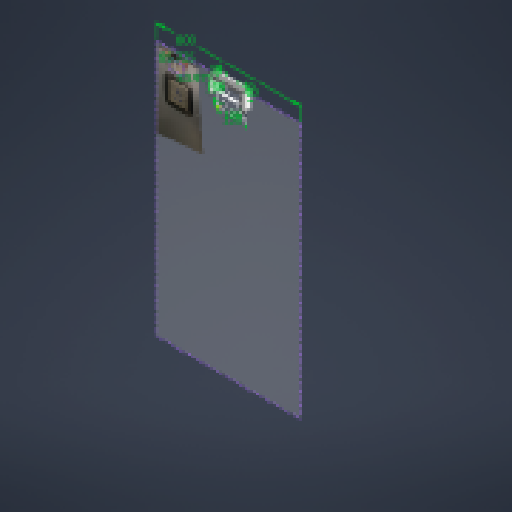
# Autodesk Inventor part: DoorButtonMount
Saved by Autodesk Inventor 2023 (Build 270158000, 158)
## iProperties
Created: 2023-12-06
Part Number: DoorButtonMount
Material: Generic
Document SubType Name: Modeling
Designer: FizzyApple12
Density: 1 g/cm^3
Appearance: Default
Author: FizzyApple12
Autodesk Inventor part; units mm, degrees
ref_plane "YZ Plane" through (0, 0, 0) normal (1, 0, 0) x (0, 1, 0)
ref_plane "XZ Plane" through (0, 0, 0) normal (0, 1, 0) x (-1, 0, 0)
ref_plane "XY Plane" through (0, 0, 0) normal (0, 0, 1) x (1, 0, 0)
sketch "Sketch1" plane through (0, 0, 0) normal (0, 0, 1) x (1, 0, 0)
  line L0 (-273.8289, 101.7521) -> (-188.1039, 101.7521) construction
  line L1 (-188.1039, 101.7521) -> (-188.1039, 47.7771) construction
  line L2 (-188.1039, 47.7771) -> (-273.8289, 47.7771) construction
  line L3 (-273.8289, 47.7771) -> (-273.8289, 101.7521) construction
  line L4 (-343.37, 152.3416) -> (456.63, 152.3416) construction
  line L5 (456.63, 152.3416) -> (456.63, -1269.8807) construction
  line L6 (456.63, -1269.8807) -> (-343.37, -1269.8807) construction
  line L7 (-343.37, -1269.8807) -> (-343.37, 152.3416) construction
  line L8 (0, 0) -> (0, 158) construction
  line L9 (0, 158) -> (158, 158) construction
  line L10 (158, 158) -> (158, 0) construction
  line L11 (158, 0) -> (0, 0) construction
  line L12 (26, 26) -> (26, 132) construction
  line L13 (26, 132) -> (132, 132) construction
  line L14 (132, 132) -> (132, 26) construction
  line L15 (132, 26) -> (26, 26) construction
  line L16 (0, 158) -> (158, 0) construction
  line L17 (26, 26) -> (132, 132) construction
  line L18 (-5, 163) -> (163, 163)
  line L19 (163, 163) -> (163, 79)
  line L20 (163, 79) -> (-5, 79)
  line L21 (-5, 79) -> (-5, 163)
  line L22 (-15, 173) -> (173, 173)
  line L23 (173, 173) -> (173, 79)
  line L24 (173, 79) -> (-15, 79)
  line L25 (-15, 79) -> (-15, 173)
  line L26 (4, 154) -> (154, 154)
  line L27 (154, 154) -> (154, 79)
  line L28 (154, 79) -> (4, 79)
  line L29 (4, 79) -> (4, 154)
  point P0 (79, 79)
  point P1 (4, 79)
  point P2 (163, 79)
  point P3 (163, 79)
  dimension "d1" = 85.725
  dimension "d2" = 53.975
  dimension "d43" = 800.0001
  dimension "d52" = 158
  dimension "d53" = 158
  dimension "d59" = 106
  dimension "d60" = 106
  dimension "d62" = 5
  dimension "d63" = 5
  dimension "d64" = 5
  dimension "d65" = 10
  dimension "d66" = 10
  dimension "d67" = 10
  dimension "d68" = 4
  dimension "d69" = 4
  dimension "d70" = 4
  constraints: 52 end point, 12 parallel, 6 perpendicular, 4 horizontal, 3 midpoint, 2 collinear, 2 vertical, 1 coincident, 2 other
  measures "d1" distance of L1.end L2.end
  measures "d2" distance of L0.end L1.end
  measures "d43" distance of L4.start L4.end
  measures "d52" distance between parallel lines of L10 L8
  measures "d53" distance between parallel lines of L9 L11
  measures "d59" distance between parallel lines of L14 L12
  measures "d60" distance between parallel lines of L13 L15
  measures "d62" distance between parallel lines of L8 L21
  measures "d63" distance between parallel lines of L10 L19
  measures "d64" distance between parallel lines of L9 L18
  measures "d65" distance between parallel lines of L25 L21
  measures "d66" distance between parallel lines of L18 L22
  measures "d67" distance between parallel lines of L19 L23
  measures "d68" distance between parallel lines of L8 L29
  measures "d69" distance between parallel lines of L9 L26
  measures "d70" distance between parallel lines of L10 L27
extrude "Extrusion1" add sketch "Sketch1" against normal blind 1 contours L21 L24 L25 L22 L23 L19 L18 | L18 L19 L20 L27 L26 L29 L21
extrude "Extrusion2" add sketch "Sketch1" along normal blind 40 contours L21 L24 L25 L22 L23 L19 L18
body "Solid1"
